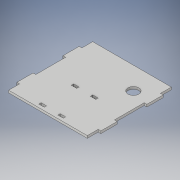
# Autodesk Inventor part: mid_floor
Saved by Autodesk Inventor 2018 (Build 220112000, 112)
## iProperties
Created: 2018-04-09
Part Number: mid_floor
Material: Generic
Document SubType Name: Modeling
Designer: guita
Density: 1 g/cm^3
Appearance: Default
Author: guita
Autodesk Inventor part; units mm, degrees
ref_plane "YZ Plane" through (0, 0, 0) normal (1, 0, 0) x (0, 1, 0)
ref_plane "XZ Plane" through (0, 0, 0) normal (0, 1, 0) x (-1, 0, 0)
ref_plane "XY Plane" through (0, 0, 0) normal (0, 0, 1) x (1, 0, 0)
sketch "Sketch1" plane through (0, 0, 0) normal (0, 1, 0) x (-1, 0, 0)
  line L0 (3.175, 0) -> (187.325, 0)
  line L1 (187.325, -196.85) -> (3.175, -196.85)
  line L2 (111.2012, -7.145) -> (111.2012, -12.7)
  line L3 (111.2012, -12.7) -> (123.9012, -12.7)
  line L4 (123.9012, -12.7) -> (123.9012, -7.145)
  line L5 (79.2988, -7.1374) -> (79.2988, -12.7)
  line L6 (79.2988, -12.7) -> (66.5988, -12.7)
  line L7 (66.5988, -12.7) -> (66.5988, -7.1374)
  line L8 (66.5988, -88.9) -> (79.2988, -88.9)
  line L9 (79.2988, -88.9) -> (79.2988, -83.3374)
  line L10 (66.5988, -83.3374) -> (66.5988, -88.9)
  line L11 (123.9012, -88.9) -> (111.2012, -88.9)
  line L12 (111.2012, -88.9) -> (111.2012, -83.3374)
  line L13 (123.9012, -83.3374) -> (123.9012, -88.9)
  line L14 (190.5, -25.4) -> (193.675, -25.4)
  line L15 (193.675, -63.5) -> (190.5, -63.5)
  line L16 (0, -25.4) -> (-3.175, -25.4)
  line L17 (-3.175, -63.5) -> (0, -63.5)
  line L18 (190.5, -171.45) -> (193.675, -171.45)
  line L19 (193.675, -133.35) -> (190.5, -133.35)
  line L20 (0, -171.45) -> (-3.175, -171.45)
  line L21 (-3.175, -133.35) -> (0, -133.35)
  line L22 (190.5, -171.45) -> (193.675, -171.45)
  line L23 (190.5, -25.4) -> (187.325, -25.4)
  line L24 (190.5, -63.5) -> (187.325, -63.5)
  line L25 (190.5, -133.35) -> (187.325, -133.35)
  line L26 (190.5, -171.45) -> (187.325, -171.45)
  line L27 (193.675, -25.4) -> (193.675, -63.5)
  line L28 (193.675, -133.35) -> (193.675, -171.45)
  line L29 (187.325, -171.45) -> (187.325, -196.85)
  line L30 (187.325, 0) -> (187.325, -25.4)
  line L31 (187.325, -63.5) -> (187.325, -133.35)
  line L32 (0, -171.45) -> (3.175, -171.45)
  line L33 (0, -133.35) -> (3.175, -133.35)
  line L34 (0, -63.5) -> (3.175, -63.5)
  line L35 (0, -25.4) -> (3.175, -25.4)
  line L36 (-3.175, -25.4) -> (-3.175, -63.5)
  line L37 (-3.175, -133.35) -> (-3.175, -171.45)
  line L38 (3.175, 0) -> (3.175, -25.4)
  line L39 (3.175, -63.5) -> (3.175, -133.35)
  line L40 (3.175, -171.45) -> (3.175, -196.85)
  line L41 (123.9012, -12.7) -> (111.2012, -12.7)
  line L42 (111.2012, -12.7) -> (111.2012, -7.145)
  line L43 (111.2012, -7.145) -> (123.9012, -7.145)
  line L44 (123.9012, -7.145) -> (123.9012, -12.7)
  line L45 (123.9012, -88.9) -> (111.2012, -88.9)
  line L46 (111.2012, -88.9) -> (111.2012, -83.3374)
  line L47 (111.2012, -83.3374) -> (123.9012, -83.3374)
  line L48 (123.9012, -83.3374) -> (123.9012, -88.9)
  line L49 (79.2988, -12.7) -> (66.5988, -12.7)
  line L50 (66.5988, -12.7) -> (66.5988, -7.1374)
  line L51 (66.5988, -7.1374) -> (79.2988, -7.1374)
  line L52 (79.2988, -7.1374) -> (79.2988, -12.7)
  line L53 (79.2988, -88.9) -> (66.5988, -88.9)
  line L54 (66.5988, -88.9) -> (66.5988, -83.3374)
  line L55 (66.5988, -83.3374) -> (79.2988, -83.3374)
  line L56 (79.2988, -83.3374) -> (79.2988, -88.9)
  point P0 (0, 0)
  dimension "d4" = 12.7
  dimension "d6" = 12.7
  dimension "d29" = 5.555
  dimension "d31" = 5.5626
  constraints: 114 end point, 26 perpendicular, 15 parallel, 8 horizontal, 1 point on line
  measures "d4" distance of L3.end L2.end
  measures "d6" distance of L5.end L6.end
  measures "d29" distance of L2.start L41.end
  measures "d31" distance of L7.end L49.end
extrude "Extrusion1" add sketch "Sketch1" along normal blind 5.5563
sketch "Sketch2" plane through (0, 5.5563, 0) normal (0, 1, 0) x (1, 0, 0)
  circle A0 centre (-39.6875, 144.4625) radius 12.7
  point P0 (0, 0)
  constraints: 1 centre point
extrude "Extrusion2" cut sketch "Sketch2" against normal blind 6.35
body "Solid1"
